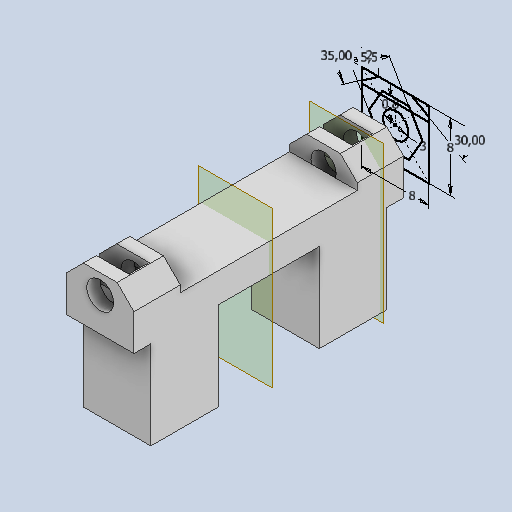
# Autodesk Inventor part: daVincihead_Sled_ToolAufnahmeBuegel
Saved by Autodesk Inventor 2024 (Build 280153000, 153)
## iProperties
Created: 2022-08-16
Part Number: daVincihead_Sled_ToolAufnahmeBuegel
Material: Generisch
Document SubType Name: Modeling
Designer: alexw
Density: 1 g/cm^3
Appearance: Vorgabe
Mass: 2.16311 g
Surface Area: 18.4939 cm^2
Volume: 2.16311 cm^3
Author: alexw
Autodesk Inventor part; units mm, degrees
ref_plane "YZ Plane" through (0, 0, 0) normal (1, 0, 0) x (0, 1, 0)
ref_plane "XZ Plane" through (0, 0, 0) normal (0, 1, 0) x (-1, 0, 0)
ref_plane "XY Plane" through (0, 0, 0) normal (0, 0, 1) x (1, 0, 0)
sketch "Skizze1" plane through (0, 0, 0) normal (0, 0, 1) x (1, 0, 0)
  line L0 (-4, 4) -> (4, 4)
  line L1 (4, 4) -> (4, -4)
  line L2 (4, -4) -> (-4, -4)
  line L3 (-4, -4) -> (-4, 4)
  line L4 (-4, 4) -> (4, -4) construction
  line L5 (4, 4) -> (-4, -4) construction
  line L6 (-4, 2.5996) -> (-2, 4)
  line L7 (1.8856, 4) -> (4, 2.7792)
  circle A0 centre (0, 0) radius 1.5
  line L8 (4, 2.3) -> (-4, 2.3)
  line L9 (0, 0) -> (0, 1.5) construction
  line L10 (3.1754, 0) -> (1.5877, -2.75)
  line L11 (1.5877, -2.75) -> (-1.5877, -2.75)
  line L12 (-1.5877, -2.75) -> (-3.1754, 0)
  line L13 (-3.1754, 0) -> (-1.5877, 2.75)
  line L14 (-1.5877, 2.75) -> (1.5877, 2.75)
  line L15 (1.5877, 2.75) -> (3.1754, 0)
  line L16 (1.5877, -2.75) -> (-4, -2.75)
  point P0 (1.8475, 2.3)
  dimension "d5" = 3
  dimension "d0" = 35
  dimension "d1" = 2
  dimension "d2" = 8
  dimension "d3" = 8
  dimension "d4" = 30
  dimension "d46" = 0.8
  dimension "d51" = 5.5
  constraints: 34 end point, 8 point on line, 3 parallel, 2 coincident, 2 midpoint, 2 perpendicular, 1 equal length, 1 horizontal, 1 vertical, 1 vertical alignment, 15 other
  measures "d0" angle of L0 L6
  measures "d1" horizontal distance of L6.end L6.start
  measures "d2" distance between parallel lines of L0 L2
  measures "d3" distance between parallel lines of L1 L3
  measures "d4" angle of L0 L7
  measures "d46" distance from line of L8 L9.end
  measures "d51" distance between parallel lines of L12 L15
extrude "Extrusion1" add sketch "Skizze1" along normal blind 38 contours L8 L13 L12 L16 L3 | L16 L11 L10 L15 L8 L1 L2 L3 | L8 L15 L10 L11 L12 L13
ref_plane "Arbeitsebene1" through (0, 0, 19) normal (0, 0, 1) x (1, 0, 0)
sketch "Skizze2" plane through (-4, -4, 0) normal (0, -1, 0) x (1, 0, 0)
  line L0 (0, 5) -> (8, 5)
  line L1 (8, 5) -> (8, 13)
  line L2 (8, 13) -> (0, 13)
  line L3 (0, 13) -> (0, 5)
  line L4 (0, 5) -> (8, 13) construction
  line L5 (8, 5) -> (0, 13) construction
  line L6 (-1.6, 19) -> (9.6, 19) construction
  line L7 (0, 0) -> (0, 38) construction
  line L8 (8, 0) -> (8, 38) construction
  line L9 (0, 33) -> (8, 33)
  line L10 (8, 33) -> (8, 25)
  line L11 (8, 25) -> (0, 25)
  line L12 (0, 25) -> (0, 33)
  line L13 (0, 33) -> (8, 25) construction
  line L14 (8, 33) -> (0, 25) construction
  line L15 (4, 0) -> (4, 19) construction
  point P0 (4, 9)
  point P1 (4, 9)
  point P2 (4, 29)
  point P3 (4, 29)
  point P4 (4, 29)
  point P5 (4, 9)
  dimension "d8" = 8
  dimension "d9" = 8
  dimension "d29" = 20
  constraints: 26 end point, 6 midpoint, 6 symmetric about line, 2 coincident, 2 collinear, 2 parallel, 2 perpendicular, 1 horizontal
  measures "d8" distance between parallel lines of L7 L8
  measures "d9" distance between parallel lines of L0 L2
  measures "d29" diameter of point (4, 9) L6
extrude "Extrusion2" add sketch "Skizze2" along normal blind 10.5
sketch "Skizze3" plane through (-4, -14.5, 0) normal (0, -1, 0) x (1, 0, 0)
  point P0 (4, 0)
  point P1 (4, 29)
  point P2 (4, 9)
hole "Bohrung1" at (0, -14.5, 29) at (0, -14.5, 9) direction (0, 1, 0) diameter 2.459 depth 8.8 tip angle 118 thread size "M3x0.5" class "6H" standard "ISO Metric profile"
sketch "Skizze5" plane through (0, 0, 19) normal (0, 0, 1) x (1, 0, 0)
  line L0 (4, -4) -> (4, 2.3) projected
  line L1 (-4, -4) -> (4, -4) projected
  line L2 (-4, 2.3) -> (-4, -4) projected
  circle A0 centre (0, 0) radius 1.5 projected
  line L3 (-4, 2.3) -> (-4, -4) projected
  line L4 (-4, -0.5) -> (4, -0.5)
  line L5 (4, -4) -> (4, 2.3) projected
  line L6 (4, 2.3) -> (-4, 2.3) projected
  point P0 (4, 2.7792)
  point P1 (-4, 2.5996)
  point P2 (1.4142, -0.5)
  point P3 (-1.4142, -0.5)
  dimension "d50" = 2.8
  constraints: 2 end point, 2 point on line, 1 perpendicular
  measures "d50" distance between parallel lines of L6 L4
ref_plane "Arbeitsebene2" through (0, 0, 29.5) normal (0, 0, 1) x (1, 0, 0)
ref_plane "Arbeitsebene3" through (0, 0, 8.5) normal (0, 0, -1) x (-1, 0, 0)
extrude "Extrusion3" cut sketch "Skizze5" along normal up to surface (10.5 mm away) contours L4 A0 L2 L6 L0 | L4 A0 picked at (0.2724, 0.086)
extrude "Extrusion4" cut sketch "Skizze5" against normal up to surface (10.5 mm away) contours L4 A0 L2 L6 L0 | L4 A0 picked at (0.2724, 0.086)
extrude "Extrusion5" add sketch "Skizze5" along normal up to surface (10.5 mm away) contours A0 L4 picked at (-0.3366, -0.703)
extrude "Extrusion6" add sketch "Skizze5" against normal up to surface (10.5 mm away) contours A0 L4 picked at (-0.3366, -0.703)
sketch "Skizze6" plane through (0, 0, 38) normal (0, 0, 1) x (1, 0, 0)
  line L0 (4, -4) -> (4, 2.3) projected
  line L1 (-4, 2.3) -> (-4, -4) projected
  line L2 (-4, -4) -> (4, -4) projected
  circle A0 centre (0, 0) radius 1.5 projected
  line L3 (4, 2.3) -> (-4, 2.3) projected
extrude "Extrusion7" cut sketch "Skizze6" against normal blind 3
sketch "Skizze7" plane through (0, 0, 0) normal (0, 0, -1) x (-1, 0, 0)
  line L0 (-4, -4) -> (-4, 2.3) projected
  line L1 (4, -4) -> (-4, -4) projected
  line L2 (4, 2.3) -> (4, -4) projected
  circle A0 centre (0, 0) radius 1.5 projected
  line L3 (-4, 2.3) -> (4, 2.3) projected
extrude "Extrusion8" cut sketch "Skizze7" against normal blind 3
chamfer "Fase2" distance 2 angle 45 4 edges at (4, 2.3, 32.25) (-4, 2.3, 32.25) (4, 2.3, 5.75) (-4, 2.3, 5.75)
ref_plane "Arbeitsebene4" through (0, 0, 5.75) normal (0, 0, -1) x (-1, 0, 0)
ref_plane "Arbeitsebene5" through (4, -4, 19) normal (0, 0, -1) x (-1, 0, 0)
extrude "Extrusion9" cut sketch "Skizze1" along normal mid plane 2.4 from surface at 5.75 contours L8 L13 L12 L16 L3 | L8 L15 L10 L11 L12 L13
mirror "Spiegeln1" about plane through (4, -4, 19) normal (0, 0, -1) of "Extrusion9"
thicken "Verdickung1" operation add thickness 0.1 both sides no extend neighbours yes toward (0.9870503, -0.1604113, 0) faces at (1.4806, -0.2406, 33.9667)
thicken "Verdickung2" operation add thickness 0.1 both sides no extend neighbours yes toward (0.9870503, -0.1604113, 0) faces at (1.4806, -0.2406, 3.5167)
equation "\"d9\" = d8"
